Autodesk Fusion 360 part; units mm, degrees
(part 6 of 7)
  spline S1657 degree 3 poles (86.8184, 41.7868) (87.2048, 41.4005) (87.7289, 41.1836) (88.2752, 41.1837) knots 0 0 0 0 1 1 1 1
  spline S1658 degree 3 poles (88.2752, 41.1837) (88.4551, 41.1837) (88.6342, 41.2074) (88.808, 41.254) knots 0 0 0 0 1 1 1 1
  spline S1659 degree 3 poles (88.808, 41.254) (88.982, 41.3005) (89.1491, 41.3696) (89.3051, 41.4596) knots 0 0 0 0 1 1 1 1
  spline S1660 degree 3 poles (89.732, 41.7868) (89.8592, 41.9141) (89.9692, 42.0576) (90.0591, 42.2136) knots 0 0 0 0 1 1 1 1
  spline S1661 degree 3 poles (102.4717, 50.3743) (102.7932, 50.3631) (103.0962, 50.5243) (103.2665, 50.7971) knots 0 0 0 0 1 1 1 1
  line L713 (100.8884, 39.3822) -> (100.8884, 39.3822)
  spline S1662 degree 3 poles (13.6891, 79.1943) (13.7972, 79.0862) (13.8906, 78.9644) (13.9671, 78.832) knots 0 0 0 0 1 1 1 1
  spline S1663 degree 3 poles (100.5907, 54.2211) (100.8269, 53.9847) (101.1474, 53.8518) (101.4816, 53.8516) knots 0 0 0 0 1 1 1 1
  spline S1664 degree 3 poles (102.7415, 55.112) (102.7415, 55.2442) (102.7208, 55.3755) (102.68, 55.5012) knots 0 0 0 0 1 1 1 1
  line L714 (101.4816, 56.3719) -> (101.4816, 56.3719)
  spline S1665 degree 3 poles (99.8394, 34.8063) (99.6692, 34.5338) (99.6572, 34.1914) (99.8078, 33.9076) knots 0 0 0 0 1 1 1 1
  spline S1666 degree 3 poles (103.2981, 51.6962) (103.1471, 51.9801) (102.8562, 52.162) (102.5348, 52.1732) knots 0 0 0 0 1 1 1 1
  spline S1667 degree 3 poles (99.6285, 38.1224) (99.6285, 37.7882) (99.7612, 37.4678) (99.9975, 37.2315) knots 0 0 0 0 1 1 1 1
  spline S1668 degree 3 poles (99.9975, 39.0133) (99.7612, 38.777) (99.6285, 38.4565) (99.6285, 38.1224) knots 0 0 0 0 1 1 1 1
  spline S1669 degree 3 poles (108.2218, 49.423) (108.0708, 49.7069) (107.7799, 49.8887) (107.4585, 49.8999) knots 0 0 0 0 1 1 1 1
  line L715 (102.5348, 52.1732) -> (101.2258, 52.2192)
  spline S1670 degree 3 poles (107.3955, 48.1011) (107.7169, 48.0899) (108.0199, 48.251) (108.1903, 48.5238) knots 0 0 0 0 1 1 1 1
  spline S1671 degree 3 poles (101.6289, 39.1414) (101.5221, 39.2192) (101.4037, 39.2798) (101.278, 39.3208) knots 0 0 0 0 1 1 1 1
  spline S1672 degree 3 poles (100.6321, 35.2295) (100.3113, 35.2399) (100.0092, 35.0786) (99.8394, 34.8063) knots 0 0 0 0 1 1 1 1
  spline S1673 degree 3 poles (102.68, 55.5012) (102.6392, 55.6269) (102.5789, 55.7455) (102.5012, 55.8526) knots 0 0 0 0 1 1 1 1
  spline S1674 degree 3 poles (101.2258, 52.2192) (100.9044, 52.2304) (100.6014, 52.0693) (100.431, 51.7965) knots 0 0 0 0 1 1 1 1
  spline S1675 degree 3 poles (88.808, 45.2336) (88.6342, 45.2802) (88.4551, 45.3038) (88.2752, 45.3038) knots 0 0 0 0 1 1 1 1
  spline S1676 degree 3 poles (102.5012, 55.8526) (102.4234, 55.9595) (102.3292, 56.0535) (102.2222, 56.1311) knots 0 0 0 0 1 1 1 1
  spline S1677 degree 3 poles (88.2752, 45.3038) (87.7288, 45.3038) (87.2048, 45.0867) (86.8184, 44.7003) knots 0 0 0 0 1 1 1 1
  spline S1678 degree 3 poles (100.3995, 50.8968) (100.5506, 50.6131) (100.8415, 50.4315) (101.1628, 50.4203) knots 0 0 0 0 1 1 1 1
  spline S1679 degree 3 poles (102.3725, 54.2211) (102.6088, 54.4574) (102.7415, 54.7779) (102.7415, 55.112) knots 0 0 0 0 1 1 1 1
  line L716 (107.4585, 49.8999) -> (106.149, 49.9459)
  spline S1680 degree 3 poles (108.1903, 48.5238) (108.3606, 48.7964) (108.3726, 49.1391) (108.2218, 49.423) knots 0 0 0 0 1 1 1 1
  spline S1681 degree 3 poles (100.431, 51.7965) (100.2605, 51.5238) (100.2485, 51.1808) (100.3995, 50.8968) knots 0 0 0 0 1 1 1 1
  line L717 (101.1628, 50.4203) -> (102.4717, 50.3743)
  line L718 (101.9416, 35.1835) -> (100.6321, 35.2295)
  spline S1682 degree 3 poles (13.3268, 79.4723) (13.4592, 79.3958) (13.581, 79.3024) (13.6891, 79.1943) knots 0 0 0 0 1 1 1 1
  spline S1683 degree 3 poles (101.7793, 37.2315) (102.0155, 37.4678) (102.1483, 37.7882) (102.1483, 38.1224) knots 0 0 0 0 1 1 1 1
  spline S1684 degree 3 poles (102.6717, 33.8079) (102.8417, 34.0802) (102.8537, 34.4225) (102.7033, 34.706) knots 0 0 0 0 1 1 1 1
  spline S1685 degree 3 poles (101.8713, 56.3104) (101.7454, 56.3512) (101.6139, 56.372) (101.4816, 56.3719) knots 0 0 0 0 1 1 1 1
  line L719 (106.0865, 48.1471) -> (107.3955, 48.1011)
  spline S1686 degree 3 poles (7.9044, 27.4543) (7.5762, 27.1261) (7.3918, 26.6809) (7.3918, 26.2166) knots 0 0 0 0 1 1 1 1
  spline S1687 degree 3 poles (10.3792, 27.4543) (10.2711, 27.5624) (10.1493, 27.6559) (10.017, 27.7323) knots 0 0 0 0 1 1 1 1
  line L720 (89.7935, 43.7174) -> (89.809, 44.6)
  spline S1688 degree 3 poles (4.2705, 32.7832) (4.5987, 32.4552) (5.0437, 32.271) (5.5077, 32.2711) knots 0 0 0 0 1 1 1 1
  spline S1689 degree 3 poles (90.0591, 42.2136) (90.149, 42.3694) (90.2182, 42.5364) (90.2647, 42.7102) knots 0 0 0 0 1 1 1 1
  spline S1690 degree 3 poles (5.5077, 32.2711) (5.9718, 32.2709) (6.417, 32.4551) (6.7453, 32.7832) knots 0 0 0 0 1 1 1 1
  spline S1691 degree 3 poles (4.2705, 35.2585) (3.9423, 34.9302) (3.7579, 34.485) (3.7579, 34.0208) knots 0 0 0 0 1 1 1 1
  spline S1692 degree 3 poles (3.7579, 34.0208) (3.7579, 33.5566) (3.9423, 33.1114) (4.2705, 32.7832) knots 0 0 0 0 1 1 1 1
  spline S1693 degree 3 poles (7.0233, 34.8957) (6.9469, 35.0283) (6.8535, 35.1502) (6.7453, 35.2585) knots 0 0 0 0 1 1 1 1
  line L721 (13.8684, 45.3834) -> (12.5636, 45.2692)
  spline S1694 degree 3 poles (14.0255, 43.5903) (14.3453, 43.6188) (14.6257, 43.8155) (14.7614, 44.1065) knots 0 0 0 0 1 1 1 1
  spline S1695 degree 3 poles (90.2647, 42.7102) (90.3114, 42.8841) (90.335, 43.0634) (90.335, 43.2435) knots 0 0 0 0 1 1 1 1
  spline S1696 degree 3 poles (10.8319, 26.6698) (10.7924, 26.8176) (10.7336, 26.9596) (10.6572, 27.092) knots 0 0 0 0 1 1 1 1
  spline S1697 degree 3 poles (11.9057, 43.8569) (12.0898, 43.5937) (12.4002, 43.4486) (12.7201, 43.4761) knots 0 0 0 0 1 1 1 1
  spline S1698 degree 3 poles (7.258, 34.0208) (7.2578, 34.1737) (7.2377, 34.3259) (7.198, 34.4735) knots 0 0 0 0 1 1 1 1
  line L722 (12.7201, 43.4761) -> (14.0255, 43.5903)
  spline S1699 degree 3 poles (9.1416, 24.4669) (9.6058, 24.4668) (10.051, 24.6512) (10.3792, 24.9795) knots 0 0 0 0 1 1 1 1
  line L723 (26.3307, 38.0412) -> (25.9297, 42.6239)
  spline S1700 degree 3 poles (10.017, 27.7323) (9.8845, 27.8087) (9.7425, 27.8675) (9.5948, 27.907) knots 0 0 0 0 1 1 1 1
  line L724 (25.9297, 42.6239) -> (28.4799, 42.8472)
  spline S1701 degree 3 poles (100.2218, 55.112) (100.2218, 54.7779) (100.3545, 54.4574) (100.5907, 54.2211) knots 0 0 0 0 1 1 1 1
  line L725 (28.438, 43.3252) -> (28.9109, 43.8884)
  spline S1702 degree 3 poles (44.1058, 40.5264) (43.9601, 40.2401) (43.978, 39.8978) (44.1528, 39.6282) knots 0 0 0 0 1 1 1 1
  spline S1703 degree 3 poles (44.1528, 39.6282) (44.3277, 39.359) (44.6327, 39.2032) (44.9533, 39.2195) knots 0 0 0 0 1 1 1 1
  spline S1704 degree 3 poles (9.5948, 27.907) (9.447, 27.9467) (9.2946, 27.9668) (9.1416, 27.9669) knots 0 0 0 0 1 1 1 1
  line L726 (90.2735, 43.7091) -> (89.7935, 43.7174)
  spline S1705 degree 3 poles (6.7453, 35.2585) (6.6371, 35.3666) (6.5151, 35.4601) (6.3826, 35.5365) knots 0 0 0 0 1 1 1 1
  spline S1706 degree 3 poles (7.198, 34.4735) (7.1585, 34.6213) (7.0998, 34.7632) (7.0233, 34.8957) knots 0 0 0 0 1 1 1 1
  spline S1707 degree 3 poles (12.5636, 45.2692) (12.2434, 45.2408) (11.9628, 45.0438) (11.8272, 44.7525) knots 0 0 0 0 1 1 1 1
  spline S1708 degree 3 poles (100.5907, 56.0029) (100.3545, 55.7666) (100.2218, 55.4462) (100.2218, 55.112) knots 0 0 0 0 1 1 1 1
  spline S1709 degree 3 poles (32.9866, 37.386) (32.6898, 37.5925) (32.3263, 37.6801) (31.9681, 37.6315) knots 0 0 0 0 1 1 1 1
  spline S1710 degree 3 poles (89.3051, 41.4596) (89.4611, 41.5496) (89.6046, 41.6595) (89.732, 41.7868) knots 0 0 0 0 1 1 1 1
  line L727 (44.9533, 39.2195) -> (46.2612, 39.2877)
  line L728 (28.9109, 43.8884) -> (33.892, 44.3246)
  line L729 (30.3738, 37.4919) -> (29.3491, 38.3053)
  line L730 (46.1672, 41.0855) -> (44.8593, 41.0168)
  line L731 (31.9681, 37.6315) -> (30.3738, 37.4919)
  spline S1711 degree 3 poles (7.3918, 26.2166) (7.3919, 25.7526) (7.5763, 25.3076) (7.9044, 24.9795) knots 0 0 0 0 1 1 1 1
  spline S1712 degree 3 poles (46.2612, 39.2877) (46.582, 39.3051) (46.8691, 39.4922) (47.0147, 39.7786) knots 0 0 0 0 1 1 1 1
  spline S1713 degree 3 poles (7.9044, 24.9795) (8.2325, 24.6514) (8.6775, 24.467) (9.1416, 24.4669) knots 0 0 0 0 1 1 1 1
  spline S1714 degree 3 poles (46.9677, 40.6762) (46.793, 40.9457) (46.4879, 41.1017) (46.1672, 41.0855) knots 0 0 0 0 1 1 1 1
  spline S1715 degree 3 poles (9.1416, 27.9669) (8.6775, 27.9668) (8.2325, 27.7824) (7.9044, 27.4543) knots 0 0 0 0 1 1 1 1
  spline S1716 degree 3 poles (33.5711, 36.5168) (33.4919, 36.8695) (33.2834, 37.1796) (32.9866, 37.386) knots 0 0 0 0 1 1 1 1
  spline S1717 degree 3 poles (6.7453, 32.7832) (7.0736, 33.1114) (7.258, 33.5566) (7.258, 34.0208) knots 0 0 0 0 1 1 1 1
  spline S1718 degree 3 poles (90.335, 43.2435) (90.3323, 43.4005) (90.3117, 43.5568) (90.2735, 43.7091) knots 0 0 0 0 1 1 1 1
  line L732 (46.1672, 41.0855) -> (46.1672, 41.0855)
  line L733 (28.4799, 42.8472) -> (28.438, 43.3252)
  spline S1719 degree 3 poles (10.3792, 24.9795) (10.7073, 25.3076) (10.8917, 25.7526) (10.8918, 26.2166) knots 0 0 0 0 1 1 1 1
  spline S1720 degree 3 poles (5.5077, 35.7706) (5.0437, 35.7706) (4.5987, 35.5864) (4.2705, 35.2585) knots 0 0 0 0 1 1 1 1
  spline S1721 degree 3 poles (10.6572, 27.092) (10.5808, 27.2244) (10.4873, 27.3462) (10.3792, 27.4543) knots 0 0 0 0 1 1 1 1
  spline S1722 degree 3 poles (6.3826, 35.5365) (6.2502, 35.6129) (6.1085, 35.6716) (5.9609, 35.7112) knots 0 0 0 0 1 1 1 1
  spline S1723 degree 3 poles (11.8272, 44.7525) (11.6917, 44.4613) (11.7217, 44.12) (11.9057, 43.8569) knots 0 0 0 0 1 1 1 1
  spline S1724 degree 3 poles (10.8918, 26.2166) (10.8918, 26.3697) (10.8716, 26.5221) (10.8319, 26.6698) knots 0 0 0 0 1 1 1 1
  line L734 (29.3491, 38.3053) -> (26.3307, 38.0412)
  line L735 (9.1416, 27.9669) -> (9.1416, 27.9669)
  spline S1725 degree 3 poles (5.9609, 35.7112) (5.8131, 35.7507) (5.6607, 35.7707) (5.5077, 35.7706) knots 0 0 0 0 1 1 1 1
  spline S1726 degree 3 poles (44.8593, 41.0168) (44.5386, 40.9994) (44.2515, 40.8125) (44.1058, 40.5264) knots 0 0 0 0 1 1 1 1
  line L736 (8.7044, 47.0397) -> (7.3995, 46.9255)
  line L737 (5.5077, 35.7706) -> (5.5077, 35.7706)
  spline S1727 degree 3 poles (9.5973, 45.7627) (9.733, 46.054) (9.7031, 46.3956) (9.5188, 46.6588) knots 0 0 0 0 1 1 1 1
  line L738 (7.5561, 45.1323) -> (8.8615, 45.2465)
  spline S1728 degree 3 poles (46.2457, 41.086) (46.5388, 41.0752) (46.8081, 40.9223) (46.9677, 40.6762) knots 0 0 0 0 1 1 1 1
  spline S1729 degree 3 poles (9.5188, 46.6588) (9.3347, 46.922) (9.0244, 47.0671) (8.7044, 47.0397) knots 0 0 0 0 1 1 1 1
  spline S1730 degree 3 poles (47.0147, 39.7786) (47.1602, 40.0648) (47.1423, 40.4068) (46.9677, 40.6762) knots 0 0 0 0 1 1 1 1
  spline S1731 degree 3 poles (6.6626, 46.4087) (6.527, 46.1174) (6.5569, 45.7759) (6.7412, 45.5126) knots 0 0 0 0 1 1 1 1
  spline S1732 degree 3 poles (7.3995, 46.9255) (7.0792, 46.8972) (6.7983, 46.7002) (6.6626, 46.4087) knots 0 0 0 0 1 1 1 1
  spline S1733 degree 3 poles (6.7412, 45.5126) (6.9255, 45.2495) (7.2361, 45.1045) (7.5561, 45.1323) knots 0 0 0 0 1 1 1 1
  spline S1734 degree 3 poles (8.8615, 45.2465) (9.1813, 45.275) (9.4617, 45.4717) (9.5973, 45.7627) knots 0 0 0 0 1 1 1 1
  spline S1735 degree 3 poles (44.9533, 39.2195) (44.6327, 39.2032) (44.3277, 39.359) (44.1528, 39.6282) knots 0 0 0 0 1 1 1 1
  line L739 (8.7044, 47.0397) -> (8.7044, 47.0397)
  spline S1736 degree 3 poles (44.1058, 40.5264) (44.2515, 40.8125) (44.5386, 40.9994) (44.8593, 41.0168) knots 0 0 0 0 1 1 1 1
  spline S1737 degree 3 poles (44.1528, 39.6282) (43.978, 39.8978) (43.9601, 40.2401) (44.1058, 40.5264) knots 0 0 0 0 1 1 1 1
  spline S1738 degree 3 poles (13.9469, 45.3865) (14.2401, 45.386) (14.5147, 45.2428) (14.6828, 45.0026) knots 0 0 0 0 1 1 1 1
  line L740 (46.2457, 41.086) -> (46.2457, 41.086)
  spline S1739 degree 3 poles (14.6828, 45.0026) (14.8671, 44.7393) (14.897, 44.3978) (14.7614, 44.1065) knots 0 0 0 0 1 1 1 1
  spline S1740 degree 3 poles (46.1672, 41.0855) (46.1934, 41.0868) (46.2196, 41.087) (46.2457, 41.086) knots 0 0 0 0 1 1 1 1
  spline S1741 degree 3 poles (12.7201, 43.4761) (12.4002, 43.4486) (12.0898, 43.5937) (11.9057, 43.8569) knots 0 0 0 0 1 1 1 1
  line L741 (44.8593, 41.0168) -> (46.1672, 41.0855)
  spline S1742 degree 3 poles (14.7614, 44.1065) (14.6257, 43.8155) (14.3453, 43.6188) (14.0255, 43.5903) knots 0 0 0 0 1 1 1 1
  line L742 (14.0255, 43.5903) -> (12.7201, 43.4761)
  spline S1743 degree 3 poles (46.9677, 40.6762) (47.1423, 40.4068) (47.1602, 40.0648) (47.0147, 39.7786) knots 0 0 0 0 1 1 1 1
  spline S1744 degree 3 poles (47.0147, 39.7786) (46.8691, 39.4922) (46.582, 39.3051) (46.2612, 39.2877) knots 0 0 0 0 1 1 1 1
  line L743 (46.2612, 39.2877) -> (44.9533, 39.2195)
  line L744 (70.0851, 82.9434) -> (68.4852, 82.9434)
  spline S1745 degree 3 poles (59.9705, 77.2166) (59.5755, 77.2167) (59.1875, 77.3208) (58.8455, 77.5184) knots 0 0 0 0 1 1 1 1
  spline S1746 degree 3 poles (71.5853, 81.6933) (71.5371, 82.0518) (71.3562, 82.3791) (71.0783, 82.6106) knots 0 0 0 0 1 1 1 1
  spline S1747 degree 3 poles (68.6185, 78.7871) (68.2321, 79.1734) (68.015, 79.6974) (68.0149, 80.2438) knots 0 0 0 0 1 1 1 1
  spline S1748 degree 3 poles (68.6185, 81.7001) (69.0048, 82.0865) (69.5289, 82.3036) (70.0753, 82.3036) knots 0 0 0 0 1 1 1 1
  spline S1749 degree 3 poles (70.3523, 89.4438) (70.5558, 89.5244) (70.7726, 89.5661) (70.9915, 89.5668) knots 0 0 0 0 1 1 1 1
  spline S1750 degree 3 poles (61.9187, 78.3416) (61.7213, 77.9997) (61.4373, 77.7158) (61.0955, 77.5184) knots 0 0 0 0 1 1 1 1
  spline S1751 degree 3 poles (58.8455, 77.5184) (58.5034, 77.7158) (58.2193, 77.9997) (58.0218, 78.3416) knots 0 0 0 0 1 1 1 1
  spline S1752 degree 3 poles (70.0753, 82.3036) (70.2552, 82.3036) (70.4343, 82.28) (70.6081, 82.2334) knots 0 0 0 0 1 1 1 1
  line L745 (56.4983, 80.0294) -> (56.548, 79.0806)
  line L746 (58.8289, 84.7578) -> (59.0021, 81.4572)
  spline S1753 degree 3 poles (59.0021, 81.4572) (59.3013, 81.6154) (59.6323, 81.7041) (59.9705, 81.7166) knots 0 0 0 0 1 1 1 1
  spline S1754 degree 3 poles (60.4707, 81.6603) (60.6351, 81.6228) (60.7947, 81.567) (60.9466, 81.4939) knots 0 0 0 0 1 1 1 1
  spline S1755 degree 3 poles (55.1796, 79.0088) (55.2126, 78.9545) (55.2414, 78.8979) (55.2659, 78.8393) knots 0 0 0 0 1 1 1 1
  spline S1756 degree 3 poles (55.2659, 78.8393) (55.3066, 78.7136) (55.3274, 78.5823) (55.3274, 78.4501) knots 0 0 0 0 1 1 1 1
  spline S1757 degree 3 poles (54.9584, 77.5592) (54.7222, 77.3228) (54.4017, 77.1899) (54.0675, 77.1897) knots 0 0 0 0 1 1 1 1
  spline S1758 degree 3 poles (55.3274, 78.4501) (55.3274, 78.116) (55.1946, 77.7955) (54.9584, 77.5592) knots 0 0 0 0 1 1 1 1
  spline S1759 degree 3 poles (70.0753, 78.1835) (69.5289, 78.1835) (69.0048, 78.4006) (68.6185, 78.7871) knots 0 0 0 0 1 1 1 1
  spline S1760 degree 3 poles (54.0675, 77.1897) (53.7333, 77.1899) (53.4128, 77.3228) (53.1766, 77.5592) knots 0 0 0 0 1 1 1 1
  spline S1761 degree 3 poles (50.5359, 78.7654) (50.546, 78.7421) (50.5556, 78.7187) (50.5649, 78.6951) knots 0 0 0 0 1 1 1 1
  spline S1762 degree 3 poles (52.8076, 78.4501) (52.8399, 78.6085) (52.9023, 78.7592) (52.9916, 78.894) knots 0 0 0 0 1 1 1 1
  spline S1763 degree 3 poles (50.5649, 78.6951) (50.6114, 78.5213) (50.6351, 78.3422) (50.6351, 78.1623) knots 0 0 0 0 1 1 1 1
  line L747 (52.9916, 78.894) -> (50.5359, 78.7654)
  spline S1764 degree 3 poles (50.6351, 78.1623) (50.6351, 77.9822) (50.6115, 77.8029) (50.5649, 77.629) knots 0 0 0 0 1 1 1 1
  line L748 (67.0651, 88.9234) -> (67.585, 89.4438)
  spline S1765 degree 3 poles (51.3416, 85.6621) (51.4403, 85.5732) (51.5707, 85.5278) (51.7033, 85.536) knots 0 0 0 0 1 1 1 1
  spline S1766 degree 3 poles (50.5649, 77.629) (50.5183, 77.455) (50.4492, 77.2879) (50.3592, 77.1319) knots 0 0 0 0 1 1 1 1
  spline S1767 degree 3 poles (50.0316, 76.7055) (49.9044, 76.5782) (49.761, 76.468) (49.6052, 76.3779) knots 0 0 0 0 1 1 1 1
  line L749 (67.585, 89.4438) -> (70.3523, 89.4438)
  line L750 (51.1255, 87.0077) -> (51.1783, 86.0088)
  spline S1768 degree 3 poles (61.7295, 80.8696) (61.8345, 80.7378) (61.9243, 80.5946) (61.9972, 80.4428) knots 0 0 0 0 1 1 1 1
  line L751 (56.1976, 85.7716) -> (56.2575, 84.6229)
  spline S1769 degree 3 poles (53.1766, 77.5592) (52.9403, 77.7955) (52.8076, 78.116) (52.8076, 78.4501) knots 0 0 0 0 1 1 1 1
  line L752 (56.548, 79.0806) -> (55.1796, 79.0088)
  line L753 (71.5853, 81.6303) -> (71.5853, 81.6933)
  line L754 (70.9915, 89.5668) -> (70.9915, 89.5668)
  line L755 (51.7033, 85.536) -> (56.1976, 85.7716)
  spline S1770 degree 3 poles (61.373, 81.2257) (61.5048, 81.1207) (61.6244, 81.0013) (61.7295, 80.8696) knots 0 0 0 0 1 1 1 1
  line L756 (57.8905, 80.1022) -> (56.4983, 80.0294)
  spline S1771 degree 3 poles (59.9705, 81.7166) (60.1388, 81.7166) (60.3066, 81.6977) (60.4707, 81.6603) knots 0 0 0 0 1 1 1 1
  spline S1772 degree 3 poles (71.1052, 82.0277) (71.261, 81.9376) (71.4043, 81.8274) (71.5315, 81.7001) knots 0 0 0 0 1 1 1 1
  spline S1773 degree 3 poles (57.7205, 79.4666) (57.7457, 79.6857) (57.803, 79.8998) (57.8905, 80.1022) knots 0 0 0 0 1 1 1 1
  spline S1774 degree 3 poles (68.0149, 80.2438) (68.0151, 80.7901) (68.2322, 81.3139) (68.6185, 81.7001) knots 0 0 0 0 1 1 1 1
  spline S1775 degree 3 poles (71.0783, 82.6106) (70.8006, 82.842) (70.4462, 82.9607) (70.0851, 82.9434) knots 0 0 0 0 1 1 1 1
  line L757 (64.5051, 88.4438) -> (67.0651, 88.4438)
  spline S1776 degree 3 poles (70.6081, 78.2538) (70.4343, 78.2072) (70.2552, 78.1835) (70.0753, 78.1835) knots 0 0 0 0 1 1 1 1
  spline S1777 degree 3 poles (71.5315, 81.7001) (71.5499, 81.6772) (71.5679, 81.6539) (71.5853, 81.6303) knots 0 0 0 0 1 1 1 1
  line L758 (68.4852, 82.9434) -> (67.5349, 83.8436)
  spline S1778 degree 3 poles (61.9972, 80.4428) (62.0703, 80.291) (62.1261, 80.1316) (62.1636, 79.9674) knots 0 0 0 0 1 1 1 1
  spline S1779 degree 3 poles (62.2205, 79.4666) (62.2204, 79.0716) (62.1163, 78.6836) (61.9187, 78.3416) knots 0 0 0 0 1 1 1 1
  line L759 (64.5051, 83.8436) -> (64.5051, 88.4438)
  spline S1780 degree 3 poles (51.1783, 86.0088) (51.1839, 85.876) (51.2428, 85.7511) (51.3416, 85.6621) knots 0 0 0 0 1 1 1 1
  line L760 (56.2575, 84.6229) -> (58.8289, 84.7578)
  spline S1781 degree 3 poles (60.9466, 81.4939) (61.0983, 81.4207) (61.2414, 81.3307) (61.373, 81.2257) knots 0 0 0 0 1 1 1 1
  spline S1782 degree 3 poles (70.6081, 82.2334) (70.7821, 82.1868) (70.9492, 82.1177) (71.1052, 82.0277) knots 0 0 0 0 1 1 1 1
  spline S1783 degree 3 poles (62.1636, 79.9674) (62.2013, 79.8031) (62.2203, 79.6351) (62.2205, 79.4666) knots 0 0 0 0 1 1 1 1
  line L761 (50.6, 87.4811) -> (51.1255, 87.0077)
  spline S1784 degree 3 poles (61.0955, 77.5184) (60.7535, 77.3208) (60.3655, 77.2167) (59.9705, 77.2166) knots 0 0 0 0 1 1 1 1
  line L762 (67.0651, 88.4438) -> (67.0651, 88.9234)
  spline S1785 degree 3 poles (58.0218, 78.3416) (57.8243, 78.6837) (57.7204, 79.0717) (57.7205, 79.4666) knots 0 0 0 0 1 1 1 1
  line L763 (67.5349, 83.8436) -> (64.5051, 83.8436)
  line L764 (91.5386, 86.3933) -> (92.03, 85.8843)
  spline S1786 degree 3 poles (46.515, 78.1623) (46.5151, 78.7085) (46.7322, 79.2323) (47.1186, 79.6185) knots 0 0 0 0 1 1 1 1
  line L765 (46.8462, 80.7751) -> (45.8504, 81.6241)
  line L766 (45.8504, 81.6241) -> (42.8242, 81.4655)
  line L767 (48.4441, 80.8588) -> (46.8462, 80.7751)
  spline S1787 degree 3 poles (92.0124, 84.8849) (92.0087, 84.7519) (92.0586, 84.623) (92.1509, 84.5273) knots 0 0 0 0 1 1 1 1
  line L768 (96.9026, 78.5483) -> (96.886, 77.5985)
  spline S1788 degree 3 poles (49.6052, 76.3779) (49.4492, 76.2879) (49.2821, 76.2188) (49.1081, 76.1722) knots 0 0 0 0 1 1 1 1
  spline S1789 degree 3 poles (49.6052, 79.9462) (49.7525, 79.8596) (49.8884, 79.7551) (50.0099, 79.6351) knots 0 0 0 0 1 1 1 1
  line L769 (99.4771, 78.5034) -> (96.9026, 78.5483)
  line L770 (99.5572, 83.1026) -> (99.4771, 78.5034)
  spline S1790 degree 3 poles (95.6277, 77.1422) (95.6277, 76.8081) (95.495, 76.4876) (95.2588, 76.2513) knots 0 0 0 0 1 1 1 1
  line L771 (93.3219, 77.661) -> (90.8673, 77.7039)
  line L772 (72.5852, 89.4438) -> (73.0849, 88.9435)
  spline S1791 degree 3 poles (50.0073, 79.6893) (49.9404, 80.0445) (49.7427, 80.3617) (49.4533, 80.5782) knots 0 0 0 0 1 1 1 1
  spline S1792 degree 3 poles (70.9915, 89.5668) (71.1445, 89.5669) (71.2969, 89.5469) (71.4447, 89.5073) knots 0 0 0 0 1 1 1 1
  line L773 (42.8242, 81.4655) -> (42.5834, 86.0595)
  spline S1793 degree 3 poles (48.5753, 80.2221) (48.7552, 80.2221) (48.9343, 80.1984) (49.1081, 80.1518) knots 0 0 0 0 1 1 1 1
  line L774 (45.607, 87.2191) -> (50.6, 87.4811)
  line L775 (50.0099, 79.6351) -> (50.0073, 79.6893)
  line L776 (73.0849, 88.9435) -> (73.0849, 87.9436)
  line L777 (69.4722, 91.2426) -> (69.4722, 91.2426)
  spline S1794 degree 3 poles (71.4447, 89.5073) (71.508, 89.4897) (71.5703, 89.4685) (71.6313, 89.4438) knots 0 0 0 0 1 1 1 1
  line L778 (78.0851, 87.4434) -> (78.0851, 86.2936)
  line L779 (80.6602, 86.2936) -> (80.6602, 81.6933)
  spline S1795 degree 3 poles (94.3679, 75.8823) (94.0335, 75.8822) (93.7129, 76.0149) (93.4764, 76.2513) knots 0 0 0 0 1 1 1 1
  spline S1796 degree 3 poles (48.5753, 76.102) (48.0289, 76.102) (47.5049, 76.3191) (47.1186, 76.7055) knots 0 0 0 0 1 1 1 1
  spline S1797 degree 3 poles (49.4533, 80.5782) (49.1639, 80.7948) (48.8037, 80.8949) (48.4441, 80.8588) knots 0 0 0 0 1 1 1 1
  spline S1798 degree 3 poles (92.1509, 84.5273) (92.2433, 84.4315) (92.3703, 84.3769) (92.5034, 84.3759) knots 0 0 0 0 1 1 1 1
  spline S1799 degree 3 poles (50.3592, 77.1319) (50.2691, 76.9761) (50.1589, 76.8327) (50.0316, 76.7055) knots 0 0 0 0 1 1 1 1
  spline S1800 degree 3 poles (47.1186, 76.7055) (46.7321, 77.0919) (46.515, 77.6159) (46.515, 78.1623) knots 0 0 0 0 1 1 1 1
  line L780 (45.1399, 86.1933) -> (45.1151, 86.6729)
  line L781 (92.5034, 84.3759) -> (97.0028, 84.2973)
  spline S1801 degree 3 poles (47.1186, 79.6185) (47.5049, 80.005) (48.0289, 80.2221) (48.5753, 80.2221) knots 0 0 0 0 1 1 1 1
  line L782 (86.5394, 86.4807) -> (91.5386, 86.3933)
  spline S1802 degree 3 poles (95.5197, 77.6223) (95.5363, 77.5928) (95.5516, 77.5626) (95.5657, 77.5318) knots 0 0 0 0 1 1 1 1
  line L783 (92.03, 85.8843) -> (92.0124, 84.8849)
  line L784 (96.886, 77.5985) -> (95.5197, 77.6223)
  spline S1803 degree 3 poles (93.1075, 77.1422) (93.139, 77.3291) (93.2123, 77.5064) (93.3219, 77.661) knots 0 0 0 0 1 1 1 1
  spline S1804 degree 3 poles (90.9283, 77.2383) (90.9284, 77.0583) (90.905, 76.879) (90.8585, 76.705) knots 0 0 0 0 1 1 1 1
  line L785 (42.5834, 86.0595) -> (45.1399, 86.1933)
  spline S1805 degree 3 poles (95.5657, 77.5318) (95.6067, 77.406) (95.6276, 77.2745) (95.6277, 77.1422) knots 0 0 0 0 1 1 1 1
  spline S1806 degree 3 poles (49.1081, 76.1722) (48.9343, 76.1256) (48.7552, 76.102) (48.5753, 76.102) knots 0 0 0 0 1 1 1 1
  line L786 (96.9827, 83.1475) -> (99.5572, 83.1026)
  spline S1807 degree 3 poles (95.2588, 76.2513) (95.0225, 76.015) (94.702, 75.8823) (94.3679, 75.8823) knots 0 0 0 0 1 1 1 1
  spline S1808 degree 3 poles (93.4764, 76.2513) (93.2402, 76.4876) (93.1075, 76.8081) (93.1075, 77.1422) knots 0 0 0 0 1 1 1 1
  spline S1809 degree 3 poles (49.1081, 80.1518) (49.2821, 80.1053) (49.4492, 80.0362) (49.6052, 79.9462) knots 0 0 0 0 1 1 1 1
  spline S1810 degree 3 poles (90.8673, 77.7039) (90.9053, 77.5516) (90.9258, 77.3953) (90.9283, 77.2383) knots 0 0 0 0 1 1 1 1
  line L787 (71.6313, 89.4438) -> (72.5852, 89.4438)
  spline S1811 degree 3 poles (77.7751, 91.0954) (75.0088, 91.2019) (72.2406, 91.251) (69.4722, 91.2426) knots 0 0 0 0 1 1 1 1
  line L788 (78.0851, 86.2936) -> (80.6602, 86.2936)
  line L789 (45.1151, 86.6729) -> (45.607, 87.2191)
  line L790 (97.0028, 84.2973) -> (96.9827, 83.1475)
  line L791 (73.5851, 87.4434) -> (78.0851, 87.4434)
  spline S1812 degree 3 poles (91.1743, 16.8741) (90.9637, 16.6315) (90.8983, 16.2952) (91.0027, 15.9914) knots 0 0 0 0 1 1 1 1
  line L792 (78.0851, 81.6933) -> (78.0851, 80.7435)
  spline S1813 degree 3 poles (76.7736, 80.6329) (76.8144, 80.5073) (76.8351, 80.376) (76.8351, 80.2438) knots 0 0 0 0 1 1 1 1
  spline S1814 degree 3 poles (76.8351, 80.2438) (76.8352, 79.9095) (76.7025, 79.5888) (76.4661, 79.3524) knots 0 0 0 0 1 1 1 1
  line L793 (74.522, 80.7435) -> (72.069, 80.7435)
  spline S1815 degree 3 poles (102.6366, 16.995) (102.4002, 17.2312) (102.2672, 17.5517) (102.2671, 17.8859) knots 0 0 0 0 1 1 1 1
  spline S1816 degree 3 poles (95.6815, 13.8587) (95.4709, 13.6162) (95.4055, 13.2799) (95.5099, 12.9761) knots 0 0 0 0 1 1 1 1
  spline S1817 degree 3 poles (72.0648, 79.7105) (72.0183, 79.5365) (71.9492, 79.3694) (71.8592, 79.2134) knots 0 0 0 0 1 1 1 1
  spline S1818 degree 3 poles (104.7874, 17.8859) (104.7874, 17.5517) (104.6547, 17.2313) (104.4184, 16.995) knots 0 0 0 0 1 1 1 1
  line L794 (78.0851, 80.7435) -> (76.7173, 80.7435)
  spline S1819 degree 3 poles (99.9122, 19.9654) (99.8223, 20.1213) (99.7123, 20.2648) (99.5851, 20.3922) knots 0 0 0 0 1 1 1 1
  line L795 (96.1879, 12.3855) -> (97.4736, 12.1353)
  spline S1820 degree 3 poles (73.2301, 87.5886) (73.3241, 87.4944) (73.4521, 87.4421) (73.5851, 87.4434) knots 0 0 0 0 1 1 1 1
  spline S1821 degree 3 poles (71.8592, 79.2134) (71.769, 79.0576) (71.6589, 78.9143) (71.5315, 78.7871) knots 0 0 0 0 1 1 1 1
  spline S1822 degree 3 poles (74.3148, 80.2438) (74.3469, 80.4234) (74.4176, 80.5939) (74.522, 80.7435) knots 0 0 0 0 1 1 1 1
  spline S1823 degree 3 poles (72.1351, 80.2438) (72.1351, 80.0637) (72.1115, 79.8845) (72.0648, 79.7105) knots 0 0 0 0 1 1 1 1
  spline S1824 degree 3 poles (104.5466, 18.6264) (104.6244, 18.5194) (104.6849, 18.4008) (104.7259, 18.275) knots 0 0 0 0 1 1 1 1
  spline S1825 degree 3 poles (103.5275, 16.626) (103.1934, 16.626) (102.8729, 16.7587) (102.6366, 16.995) knots 0 0 0 0 1 1 1 1
  spline S1826 degree 3 poles (72.069, 80.7435) (72.1114, 80.5803) (72.1336, 80.4125) (72.1351, 80.2438) knots 0 0 0 0 1 1 1 1
  spline S1827 degree 3 poles (96.5315, 14.1523) (96.2161, 14.2132) (95.8921, 14.1013) (95.6815, 13.8587) knots 0 0 0 0 1 1 1 1
  spline S1828 degree 3 poles (97.4736, 12.1353) (97.7888, 12.075) (98.1123, 12.187) (98.3226, 12.4294) knots 0 0 0 0 1 1 1 1
  spline S1829 degree 3 poles (99.5851, 20.3922) (99.4577, 20.5194) (99.3142, 20.6294) (99.1583, 20.7193) knots 0 0 0 0 1 1 1 1
  spline S1830 degree 3 poles (98.4937, 13.3115) (98.3896, 13.6148) (98.1319, 13.8399) (97.8173, 13.9022) knots 0 0 0 0 1 1 1 1
  spline S1831 degree 3 poles (91.0027, 15.9914) (91.1071, 15.6877) (91.3655, 15.4626) (91.6807, 15.4008) knots 0 0 0 0 1 1 1 1
  line L796 (98.1283, 20.9953) -> (98.1283, 20.9953)
  line L797 (91.6807, 15.4008) -> (92.9664, 15.1507)
  spline S1832 degree 3 poles (99.1583, 20.7193) (99.0024, 20.8093) (98.8355, 20.8784) (98.6616, 20.925) knots 0 0 0 0 1 1 1 1
  spline S1833 degree 3 poles (93.9891, 16.3273) (93.8843, 16.6312) (93.6255, 16.8561) (93.31, 16.9175) knots 0 0 0 0 1 1 1 1
  spline S1834 degree 3 poles (104.268, 18.9055) (104.3749, 18.8276) (104.4689, 18.7335) (104.5466, 18.6264) knots 0 0 0 0 1 1 1 1
  spline S1835 degree 3 poles (76.7173, 80.7435) (76.7378, 80.7076) (76.7566, 80.6707) (76.7736, 80.6329) knots 0 0 0 0 1 1 1 1
  spline S1836 degree 3 poles (104.4184, 16.995) (104.1821, 16.7587) (103.8616, 16.626) (103.5275, 16.626) knots 0 0 0 0 1 1 1 1
  spline S1837 degree 3 poles (98.3226, 12.4294) (98.5329, 12.6719) (98.598, 13.008) (98.4937, 13.3115) knots 0 0 0 0 1 1 1 1
  spline S1838 degree 3 poles (76.4661, 79.3524) (76.2298, 79.1162) (75.9094, 78.9834) (75.5752, 78.9834) knots 0 0 0 0 1 1 1 1
  spline S1839 degree 3 poles (92.0238, 17.1676) (91.7085, 17.2283) (91.3848, 17.1164) (91.1743, 16.8741) knots 0 0 0 0 1 1 1 1
  spline S1840 degree 3 poles (73.0849, 87.9436) (73.0836, 87.8106) (73.136, 87.6826) (73.2301, 87.5886) knots 0 0 0 0 1 1 1 1
  spline S1841 degree 3 poles (74.6843, 79.3524) (74.4477, 79.5887) (74.3148, 79.9094) (74.3148, 80.2438) knots 0 0 0 0 1 1 1 1
  spline S1842 degree 3 poles (98.6616, 20.925) (98.4877, 20.9716) (98.3084, 20.9952) (98.1283, 20.9953) knots 0 0 0 0 1 1 1 1
  spline S1843 degree 3 poles (104.7259, 18.275) (104.7666, 18.1493) (104.7874, 18.018) (104.7874, 17.8859) knots 0 0 0 0 1 1 1 1
  spline S1844 degree 3 poles (75.5752, 78.9834) (75.2411, 78.9834) (74.9206, 79.1162) (74.6843, 79.3524) knots 0 0 0 0 1 1 1 1
  spline S1845 degree 3 poles (71.1052, 78.4594) (70.9492, 78.3694) (70.7821, 78.3003) (70.6081, 78.2538) knots 0 0 0 0 1 1 1 1
  spline S1846 degree 3 poles (95.5099, 12.9761) (95.6143, 12.6723) (95.8727, 12.4472) (96.1879, 12.3855) knots 0 0 0 0 1 1 1 1
  line L798 (97.8173, 13.9022) -> (96.5315, 14.1523)
  line L799 (80.6602, 81.6933) -> (78.0851, 81.6933)
  spline S1847 degree 3 poles (71.5315, 78.7871) (71.4043, 78.6597) (71.261, 78.5496) (71.1052, 78.4594) knots 0 0 0 0 1 1 1 1
  spline S1848 degree 3 poles (91.4693, 19.985) (91.4692, 19.6507) (91.6019, 19.33) (91.8383, 19.0936) knots 0 0 0 0 1 1 1 1
  spline S1849 degree 3 poles (92.9664, 15.1507) (93.2821, 15.0892) (93.6065, 15.2009) (93.8175, 15.4437) knots 0 0 0 0 1 1 1 1
  spline S1850 degree 3 poles (92.7292, 18.7246) (92.8615, 18.7247) (92.993, 18.7456) (93.1188, 18.7866) knots 0 0 0 0 1 1 1 1
  line L800 (39.3118, 20.7818) -> (86.2118, 20.7818)
  spline S1851 degree 3 poles (91.8383, 19.0936) (92.0746, 18.8573) (92.3951, 18.7246) (92.7292, 18.7246) knots 0 0 0 0 1 1 1 1
  line L801 (86.2118, 38.372) -> (42.5183, 38.372)
  spline S1852 degree 3 poles (93.1188, 18.7866) (93.2446, 18.8274) (93.3632, 18.8877) (93.4702, 18.9654) knots 0 0 0 0 1 1 1 1
  spline S1853 degree 3 poles (92.7292, 21.2449) (92.3951, 21.2449) (92.0746, 21.1121) (91.8383, 20.8759) knots 0 0 0 0 1 1 1 1
  line L802 (42.5183, 38.372) -> (42.6113, 37.3074)
  spline S1854 degree 3 poles (93.4702, 18.9654) (93.5771, 19.0431) (93.6711, 19.1371) (93.7488, 19.2439) knots 0 0 0 0 1 1 1 1
  line L803 (92.7292, 21.2449) -> (92.7292, 21.2449)
  spline S1855 degree 3 poles (93.9276, 19.5953) (93.9686, 19.7212) (93.9895, 19.8527) (93.9896, 19.985) knots 0 0 0 0 1 1 1 1
  line L804 (42.6113, 37.3074) -> (40.0461, 37.0832)
  line L805 (40.0461, 37.0832) -> (40.1293, 36.137)
  line L806 (96.5315, 14.1523) -> (97.8173, 13.9022)
  spline S1856 degree 3 poles (98.3226, 12.4294) (98.1123, 12.187) (97.7888, 12.075) (97.4736, 12.1353) knots 0 0 0 0 1 1 1 1
  line L807 (86.2118, 20.7818) -> (86.2118, 38.372)
  line L808 (39.3118, 36.0657) -> (39.3118, 20.7818)
  spline S1857 degree 3 poles (93.9896, 19.985) (93.9894, 20.1171) (93.9685, 20.2485) (93.9276, 20.3741) knots 0 0 0 0 1 1 1 1
  line L809 (40.1293, 36.137) -> (39.3118, 36.0657)
  spline S1858 degree 3 poles (93.9276, 20.3741) (93.8868, 20.4999) (93.8264, 20.6185) (93.7488, 20.7255) knots 0 0 0 0 1 1 1 1
  spline S1859 degree 3 poles (93.7488, 19.2439) (93.8264, 19.351) (93.8868, 19.4696) (93.9276, 19.5953) knots 0 0 0 0 1 1 1 1
  spline S1860 degree 3 poles (91.8383, 20.8759) (91.602, 20.6396) (91.4693, 20.3191) (91.4693, 19.985) knots 0 0 0 0 1 1 1 1
  line L810 (93.31, 16.9175) -> (92.0238, 17.1676)
  spline S1861 degree 3 poles (97.8173, 13.9022) (98.1319, 13.8399) (98.3896, 13.6148) (98.4937, 13.3115) knots 0 0 0 0 1 1 1 1
  spline S1862 degree 3 poles (96.3755, 14.1683) (96.4279, 14.1675) (96.4801, 14.1621) (96.5315, 14.1523) knots 0 0 0 0 1 1 1 1
  spline S1863 degree 3 poles (98.4937, 13.3115) (98.598, 13.008) (98.5329, 12.6719) (98.3226, 12.4294) knots 0 0 0 0 1 1 1 1
  line L811 (97.4736, 12.1353) -> (96.1879, 12.3855)
  spline S1864 degree 3 poles (93.7488, 20.7255) (93.6711, 20.8324) (93.5771, 20.9264) (93.4702, 21.004) knots 0 0 0 0 1 1 1 1
  spline S1865 degree 3 poles (93.1188, 21.1834) (92.993, 21.2242) (92.8615, 21.2449) (92.7292, 21.2449) knots 0 0 0 0 1 1 1 1
  spline S1866 degree 3 poles (93.4702, 21.004) (93.3632, 21.0819) (93.2447, 21.1424) (93.1188, 21.1834) knots 0 0 0 0 1 1 1 1
  spline S1867 degree 3 poles (93.8175, 15.4437) (94.0285, 15.6864) (94.0939, 16.0233) (93.9891, 16.3273) knots 0 0 0 0 1 1 1 1
  spline S1868 degree 3 poles (91.6807, 15.4008) (91.3655, 15.4626) (91.1071, 15.6877) (91.0027, 15.9914) knots 0 0 0 0 1 1 1 1
  spline S1869 degree 3 poles (70.9848, 20.217) (70.837, 20.2567) (70.6846, 20.2769) (70.5316, 20.277) knots 0 0 0 0 1 1 1 1
  spline S1870 degree 3 poles (68.7818, 18.5267) (68.7819, 18.0626) (68.9663, 17.6176) (69.2945, 17.2895) knots 0 0 0 0 1 1 1 1
  line L812 (91.8677, 17.1836) -> (91.8677, 17.1836)
  line L813 (92.9664, 15.1507) -> (91.6807, 15.4008)
  spline S1871 degree 3 poles (72.2219, 18.9799) (72.1824, 19.1275) (72.1236, 19.2692) (72.0473, 19.4016) knots 0 0 0 0 1 1 1 1
  spline S1872 degree 3 poles (71.4065, 20.0423) (71.2741, 20.1187) (71.1324, 20.1775) (70.9848, 20.217) knots 0 0 0 0 1 1 1 1
  line L814 (32.1334, 28.1096) -> (33.4383, 28.2238)
  spline S1873 degree 3 poles (70.5316, 16.7769) (70.9958, 16.7769) (71.441, 16.9613) (71.7692, 17.2895) knots 0 0 0 0 1 1 1 1
  spline S1874 degree 3 poles (93.8175, 15.4437) (93.6065, 15.2009) (93.2821, 15.0892) (92.9664, 15.1507) knots 0 0 0 0 1 1 1 1
  spline S1875 degree 3 poles (33.4383, 28.2238) (33.7581, 28.2523) (34.0385, 28.449) (34.1741, 28.74) knots 0 0 0 0 1 1 1 1
  spline S1876 degree 3 poles (95.6815, 13.8587) (95.8558, 14.0593) (96.1098, 14.1726) (96.3755, 14.1683) knots 0 0 0 0 1 1 1 1
  spline S1877 degree 3 poles (95.5099, 12.9761) (95.4055, 13.2799) (95.4709, 13.6162) (95.6815, 13.8587) knots 0 0 0 0 1 1 1 1
  line L815 (92.0238, 17.1676) -> (93.31, 16.9175)
  spline S1878 degree 3 poles (31.2394, 29.3865) (31.1034, 29.0951) (31.1332, 28.7534) (31.3175, 28.4899) knots 0 0 0 0 1 1 1 1
  spline S1879 degree 3 poles (72.0473, 19.4016) (71.9708, 19.5341) (71.8774, 19.6561) (71.7692, 19.7643) knots 0 0 0 0 1 1 1 1
  line L816 (33.2817, 30.0169) -> (33.2817, 30.0169)
  line L817 (33.2817, 30.0169) -> (31.9763, 29.9027)
  spline S1880 degree 3 poles (93.9891, 16.3273) (94.0939, 16.0233) (94.0285, 15.6864) (93.8175, 15.4437) knots 0 0 0 0 1 1 1 1
  spline S1881 degree 3 poles (91.0027, 15.9914) (90.8983, 16.2952) (90.9637, 16.6315) (91.1743, 16.8741) knots 0 0 0 0 1 1 1 1
  spline S1882 degree 3 poles (70.5316, 20.277) (70.0676, 20.2769) (69.6226, 20.0925) (69.2945, 19.7643) knots 0 0 0 0 1 1 1 1
  spline S1883 degree 3 poles (69.2945, 19.7643) (68.9662, 19.4361) (68.7818, 18.9909) (68.7818, 18.5267) knots 0 0 0 0 1 1 1 1
  line L818 (70.5316, 20.277) -> (70.5316, 20.277)
  spline S1884 degree 3 poles (26.1545, 30.1461) (26.3388, 29.883) (26.6493, 29.738) (26.9694, 29.7658) knots 0 0 0 0 1 1 1 1
  spline S1885 degree 3 poles (26.0759, 31.0422) (25.9403, 30.7509) (25.9702, 30.4094) (26.1545, 30.1461) knots 0 0 0 0 1 1 1 1
  spline S1886 degree 3 poles (28.2742, 29.88) (28.5941, 29.9085) (28.8745, 30.1052) (29.0101, 30.3962) knots 0 0 0 0 1 1 1 1
  spline S1887 degree 3 poles (29.0101, 30.3962) (29.1459, 30.6874) (29.1162, 31.029) (28.9321, 31.2923) knots 0 0 0 0 1 1 1 1
  spline S1888 degree 3 poles (28.9321, 31.2923) (28.748, 31.5555) (28.4376, 31.7006) (28.1177, 31.6732) knots 0 0 0 0 1 1 1 1
  spline S1889 degree 3 poles (103.5275, 19.1458) (103.6596, 19.1458) (103.7909, 19.125) (103.9166, 19.0843) knots 0 0 0 0 1 1 1 1
  spline S1890 degree 3 poles (17.3684, 49.8953) (17.6047, 49.659) (17.9252, 49.5263) (18.2593, 49.5263) knots 0 0 0 0 1 1 1 1
  spline S1891 degree 3 poles (24.3417, 52.2874) (24.1054, 52.0511) (23.9727, 51.7306) (23.9727, 51.3965) knots 0 0 0 0 1 1 1 1
  spline S1892 degree 3 poles (26.8123, 31.559) (26.4922, 31.5305) (26.2115, 31.3336) (26.0759, 31.0422) knots 0 0 0 0 1 1 1 1
  spline S1893 degree 3 poles (31.9763, 29.9027) (31.6561, 29.8746) (31.3752, 29.6778) (31.2394, 29.3865) knots 0 0 0 0 1 1 1 1
  spline S1894 degree 3 poles (71.7692, 17.2895) (72.0974, 17.6176) (72.2818, 18.0626) (72.2819, 18.5267) knots 0 0 0 0 1 1 1 1
  spline S1895 degree 3 poles (69.2945, 17.2895) (69.6226, 16.9614) (70.0676, 16.777) (70.5316, 16.7769) knots 0 0 0 0 1 1 1 1
  spline S1896 degree 3 poles (31.3175, 28.4899) (31.5019, 28.2264) (31.813, 28.0814) (32.1334, 28.1096) knots 0 0 0 0 1 1 1 1
  spline S1897 degree 3 poles (34.1741, 28.74) (34.3099, 29.0312) (34.2802, 29.3727) (34.0961, 29.6361) knots 0 0 0 0 1 1 1 1
  line L819 (96.3755, 14.1683) -> (96.3755, 14.1683)
  spline S1898 degree 3 poles (34.0961, 29.6361) (33.912, 29.8992) (33.6017, 30.0444) (33.2817, 30.0169) knots 0 0 0 0 1 1 1 1
  line L820 (28.1177, 31.6732) -> (28.1177, 31.6732)
  spline S1899 degree 3 poles (103.9166, 19.0843) (104.0424, 19.0435) (104.161, 18.9831) (104.268, 18.9055) knots 0 0 0 0 1 1 1 1
  spline S1900 degree 3 poles (18.2593, 49.5263) (18.5935, 49.5263) (18.9139, 49.659) (19.1502, 49.8953) knots 0 0 0 0 1 1 1 1
  spline S1901 degree 3 poles (19.5192, 50.7867) (19.5192, 50.9188) (19.4985, 51.0502) (19.4577, 51.1758) knots 0 0 0 0 1 1 1 1
  line L821 (26.9694, 29.7658) -> (28.2742, 29.88)
  line L822 (28.1177, 31.6732) -> (26.8123, 31.559)
  line L823 (19.3513, 51.3841) -> (17.1674, 51.1929)
  spline S1902 degree 3 poles (25.2326, 52.6564) (24.8984, 52.6564) (24.578, 52.5237) (24.3417, 52.2874) knots 0 0 0 0 1 1 1 1
  spline S1903 degree 3 poles (19.4577, 51.1758) (19.4288, 51.2484) (19.3931, 51.3181) (19.3513, 51.3841) knots 0 0 0 0 1 1 1 1
  spline S1904 degree 3 poles (23.9727, 51.3965) (23.9727, 51.0624) (24.1054, 50.7419) (24.3417, 50.5056) knots 0 0 0 0 1 1 1 1
  spline S1905 degree 3 poles (24.3417, 50.5056) (24.578, 50.2693) (24.8984, 50.1366) (25.2326, 50.1366) knots 0 0 0 0 1 1 1 1
  spline S1906 degree 3 poles (25.6217, 50.1981) (25.7475, 50.2389) (25.8661, 50.2993) (25.9731, 50.3769) knots 0 0 0 0 1 1 1 1
  spline S1907 degree 3 poles (19.1502, 49.8953) (19.3866, 50.1317) (19.5194, 50.4524) (19.5192, 50.7867) knots 0 0 0 0 1 1 1 1
  spline S1908 degree 3 poles (25.9731, 50.3769) (26.08, 50.4547) (26.174, 50.5489) (26.2516, 50.656) knots 0 0 0 0 1 1 1 1
  spline S1909 degree 3 poles (72.2819, 18.5267) (72.2818, 18.6797) (72.2616, 18.8321) (72.2219, 18.9799) knots 0 0 0 0 1 1 1 1
  spline S1910 degree 3 poles (25.2326, 50.1366) (25.3647, 50.1366) (25.496, 50.1573) (25.6217, 50.1981) knots 0 0 0 0 1 1 1 1
  spline S1911 degree 3 poles (26.2516, 50.656) (26.3295, 50.763) (26.39, 50.8816) (26.4309, 51.0074) knots 0 0 0 0 1 1 1 1
  spline S1912 degree 3 poles (26.4924, 51.3965) (26.4925, 51.5288) (26.4718, 51.6603) (26.4309, 51.7861) knots 0 0 0 0 1 1 1 1
  spline S1913 degree 3 poles (26.2516, 52.137) (26.174, 52.2441) (26.08, 52.3382) (25.9731, 52.4161) knots 0 0 0 0 1 1 1 1
  spline S1914 degree 3 poles (93.31, 16.9175) (93.6255, 16.8561) (93.8843, 16.6312) (93.9891, 16.3273) knots 0 0 0 0 1 1 1 1
  spline S1915 degree 3 poles (26.4309, 51.0074) (26.4717, 51.1331) (26.4925, 51.2644) (26.4924, 51.3965) knots 0 0 0 0 1 1 1 1
  spline S1916 degree 3 poles (91.1743, 16.8741) (91.3484, 17.0745) (91.6022, 17.1878) (91.8677, 17.1836) knots 0 0 0 0 1 1 1 1
  spline S1917 degree 3 poles (96.1879, 12.3855) (95.8727, 12.4472) (95.6143, 12.6723) (95.5099, 12.9761) knots 0 0 0 0 1 1 1 1
  spline S1918 degree 3 poles (91.8677, 17.1836) (91.9201, 17.1828) (91.9724, 17.1775) (92.0238, 17.1676) knots 0 0 0 0 1 1 1 1
  spline S1919 degree 3 poles (71.7692, 19.7643) (71.661, 19.8725) (71.539, 19.9659) (71.4065, 20.0423) knots 0 0 0 0 1 1 1 1
  spline S1920 degree 3 poles (61.0955, 77.5184) (61.4373, 77.7158) (61.7213, 77.9997) (61.9187, 78.3416) knots 0 0 0 0 1 1 1 1
  spline S1921 degree 3 poles (61.9972, 80.4428) (61.9243, 80.5946) (61.8345, 80.7378) (61.7295, 80.8696) knots 0 0 0 0 1 1 1 1
  spline S1922 degree 3 poles (55.2659, 78.8393) (55.2414, 78.8979) (55.2126, 78.9545) (55.1796, 79.0088) knots 0 0 0 0 1 1 1 1
  spline S1923 degree 3 poles (49.1081, 80.1518) (48.9343, 80.1984) (48.7552, 80.2221) (48.5753, 80.2221) knots 0 0 0 0 1 1 1 1
  spline S1924 degree 3 poles (25.6217, 52.5949) (25.496, 52.6356) (25.3647, 52.6564) (25.2326, 52.6564) knots 0 0 0 0 1 1 1 1
  spline S1925 degree 3 poles (61.373, 43.1257) (61.2414, 43.2308) (61.0983, 43.3207) (60.9466, 43.3939) knots 0 0 0 0 1 1 1 1
  line L824 (59.9705, 43.6166) -> (59.9705, 43.6166)
  spline S1926 degree 3 poles (25.9731, 52.4161) (25.8661, 52.4937) (25.7475, 52.5541) (25.6217, 52.5949) knots 0 0 0 0 1 1 1 1
  spline S1927 degree 3 poles (60.4707, 81.6603) (60.3066, 81.6977) (60.1388, 81.7166) (59.9705, 81.7166) knots 0 0 0 0 1 1 1 1
  spline S1928 degree 3 poles (59.9705, 81.7166) (59.6323, 81.7041) (59.3013, 81.6154) (59.0021, 81.4572) knots 0 0 0 0 1 1 1 1
  spline S1929 degree 3 poles (47.1186, 79.6185) (46.7322, 79.2323) (46.5151, 78.7085) (46.515, 78.1623) knots 0 0 0 0 1 1 1 1
  spline S1930 degree 3 poles (61.0955, 39.4184) (61.4373, 39.6159) (61.7213, 39.8998) (61.9187, 40.2416) knots 0 0 0 0 1 1 1 1
  spline S1931 degree 3 poles (58.8455, 39.4184) (59.1875, 39.2208) (59.5755, 39.1167) (59.9705, 39.1166) knots 0 0 0 0 1 1 1 1
  spline S1932 degree 3 poles (62.2205, 41.3666) (62.2203, 41.5351) (62.2013, 41.7031) (62.1636, 41.8674) knots 0 0 0 0 1 1 1 1
  spline S1933 degree 3 poles (57.7205, 41.3666) (57.7204, 40.9717) (57.8243, 40.5837) (58.0218, 40.2416) knots 0 0 0 0 1 1 1 1
  spline S1934 degree 3 poles (60.9466, 43.3939) (60.7947, 43.467) (60.6351, 43.5228) (60.4707, 43.5603) knots 0 0 0 0 1 1 1 1
  spline S1935 degree 3 poles (62.1636, 79.9674) (62.1261, 80.1316) (62.0703, 80.291) (61.9972, 80.4428) knots 0 0 0 0 1 1 1 1
  spline S1936 degree 3 poles (60.4707, 43.5603) (60.3066, 43.5977) (60.1388, 43.6166) (59.9705, 43.6166) knots 0 0 0 0 1 1 1 1
  spline S1937 degree 3 poles (26.4309, 51.7861) (26.3899, 51.9118) (26.3294, 52.0302) (26.2516, 52.137) knots 0 0 0 0 1 1 1 1
  spline S1938 degree 3 poles (62.2205, 79.4666) (62.2203, 79.6351) (62.2013, 79.8031) (62.1636, 79.9674) knots 0 0 0 0 1 1 1 1
  spline S1939 degree 3 poles (52.8076, 78.4501) (52.8076, 78.116) (52.9403, 77.7955) (53.1766, 77.5592) knots 0 0 0 0 1 1 1 1
  spline S1940 degree 3 poles (55.3274, 78.4501) (55.3274, 78.5823) (55.3066, 78.7136) (55.2659, 78.8393) knots 0 0 0 0 1 1 1 1
  spline S1941 degree 3 poles (50.0099, 79.6351) (49.8884, 79.7551) (49.7525, 79.8596) (49.6052, 79.9462) knots 0 0 0 0 1 1 1 1
  spline S1942 degree 3 poles (47.1186, 76.7055) (47.5049, 76.3191) (48.0289, 76.102) (48.5753, 76.102) knots 0 0 0 0 1 1 1 1
  spline S1943 degree 3 poles (49.1081, 76.1722) (49.2821, 76.2188) (49.4492, 76.2879) (49.6052, 76.3779) knots 0 0 0 0 1 1 1 1
  spline S1944 degree 3 poles (49.6052, 79.9462) (49.4492, 80.0362) (49.2821, 80.1053) (49.1081, 80.1518) knots 0 0 0 0 1 1 1 1
  spline S1945 degree 3 poles (48.5753, 76.102) (48.7552, 76.102) (48.9343, 76.1256) (49.1081, 76.1722) knots 0 0 0 0 1 1 1 1
  spline S1946 degree 3 poles (52.9916, 78.894) (52.9023, 78.7592) (52.8399, 78.6085) (52.8076, 78.4501) knots 0 0 0 0 1 1 1 1
  spline S1947 degree 3 poles (50.0316, 76.7055) (50.1589, 76.8327) (50.2691, 76.9761) (50.3592, 77.1319) knots 0 0 0 0 1 1 1 1
  spline S1948 degree 3 poles (59.9705, 39.1166) (60.3655, 39.1167) (60.7535, 39.2208) (61.0955, 39.4184) knots 0 0 0 0 1 1 1 1
  spline S1949 degree 3 poles (54.0675, 77.1897) (54.4017, 77.1899) (54.7222, 77.3228) (54.9584, 77.5592) knots 0 0 0 0 1 1 1 1
  spline S1950 degree 3 poles (57.7205, 79.4666) (57.7204, 79.0717) (57.8243, 78.6837) (58.0218, 78.3416) knots 0 0 0 0 1 1 1 1
  spline S1951 degree 3 poles (58.8455, 77.5184) (59.1875, 77.3208) (59.5755, 77.2167) (59.9705, 77.2166) knots 0 0 0 0 1 1 1 1
  spline S1952 degree 3 poles (58.8455, 43.3153) (58.5034, 43.1178) (58.2193, 42.8337) (58.0218, 42.4916) knots 0 0 0 0 1 1 1 1
  spline S1953 degree 3 poles (53.1766, 77.5592) (53.4128, 77.3228) (53.7333, 77.1899) (54.0675, 77.1897) knots 0 0 0 0 1 1 1 1
  spline S1954 degree 3 poles (46.515, 78.1623) (46.515, 77.6159) (46.7321, 77.0919) (47.1186, 76.7055) knots 0 0 0 0 1 1 1 1
  spline S1955 degree 3 poles (60.9466, 81.4939) (60.7947, 81.567) (60.6351, 81.6228) (60.4707, 81.6603) knots 0 0 0 0 1 1 1 1
  spline S1956 degree 3 poles (62.1636, 41.8674) (62.1262, 42.0317) (62.0704, 42.1914) (61.9972, 42.3433) knots 0 0 0 0 1 1 1 1
  spline S1957 degree 3 poles (61.9972, 42.3433) (61.9242, 42.495) (61.8344, 42.638) (61.7295, 42.7696) knots 0 0 0 0 1 1 1 1
  spline S1958 degree 3 poles (58.0218, 78.3416) (58.2193, 77.9997) (58.5034, 77.7158) (58.8455, 77.5184) knots 0 0 0 0 1 1 1 1
  spline S1959 degree 3 poles (48.5753, 80.2221) (48.0289, 80.2221) (47.5049, 80.005) (47.1186, 79.6185) knots 0 0 0 0 1 1 1 1
  spline S1960 degree 3 poles (49.6052, 76.3779) (49.761, 76.468) (49.9044, 76.5782) (50.0316, 76.7055) knots 0 0 0 0 1 1 1 1
  spline S1961 degree 3 poles (61.9187, 78.3416) (62.1163, 78.6836) (62.2204, 79.0716) (62.2205, 79.4666) knots 0 0 0 0 1 1 1 1
  spline S1962 degree 3 poles (61.7295, 80.8696) (61.6244, 81.0013) (61.5048, 81.1207) (61.373, 81.2257) knots 0 0 0 0 1 1 1 1
  spline S1963 degree 3 poles (58.0218, 42.4916) (57.8243, 42.1496) (57.7204, 41.7616) (57.7205, 41.3666) knots 0 0 0 0 1 1 1 1
  line L825 (25.2326, 52.6564) -> (25.2326, 52.6564)
  line L826 (59.0021, 81.4572) -> (59.0698, 80.1642)
  spline S1964 degree 3 poles (54.9584, 77.5592) (55.1946, 77.7955) (55.3274, 78.116) (55.3274, 78.4501) knots 0 0 0 0 1 1 1 1
  spline S1965 degree 3 poles (50.3592, 77.1319) (50.4492, 77.2879) (50.5183, 77.455) (50.5649, 77.629) knots 0 0 0 0 1 1 1 1
  spline S1966 degree 3 poles (50.5649, 77.629) (50.6115, 77.8029) (50.6351, 77.9822) (50.6351, 78.1623) knots 0 0 0 0 1 1 1 1
  spline S1967 degree 3 poles (43.0826, 79.1343) (42.7485, 79.1343) (42.428, 79.0016) (42.1917, 78.7654) knots 0 0 0 0 1 1 1 1
  line L827 (50.5359, 78.7654) -> (50.0569, 78.7406)
  line L828 (50.0569, 78.7406) -> (50.0099, 79.6351)
  line L829 (59.0698, 80.1642) -> (57.8905, 80.1022)
  spline S1968 degree 3 poles (59.9705, 43.6166) (59.5755, 43.6167) (59.1875, 43.5128) (58.8455, 43.3153) knots 0 0 0 0 1 1 1 1
  spline S1969 degree 3 poles (58.0218, 40.2416) (58.2193, 39.8997) (58.5034, 39.6158) (58.8455, 39.4184) knots 0 0 0 0 1 1 1 1
  line L830 (55.1796, 79.0088) -> (52.9916, 78.894)
  spline S1970 degree 3 poles (59.9705, 77.2166) (60.3655, 77.2167) (60.7535, 77.3208) (61.0955, 77.5184) knots 0 0 0 0 1 1 1 1
  spline S1971 degree 3 poles (50.6351, 78.1623) (50.6351, 78.3422) (50.6114, 78.5213) (50.5649, 78.6951) knots 0 0 0 0 1 1 1 1
  spline S1972 degree 3 poles (50.5649, 78.6951) (50.5556, 78.7187) (50.546, 78.7421) (50.5359, 78.7654) knots 0 0 0 0 1 1 1 1
  spline S1973 degree 3 poles (61.7295, 42.7696) (61.6244, 42.9013) (61.5048, 43.0207) (61.373, 43.1257) knots 0 0 0 0 1 1 1 1
  spline S1974 degree 3 poles (61.9187, 40.2416) (62.1163, 40.5836) (62.2204, 40.9716) (62.2205, 41.3666) knots 0 0 0 0 1 1 1 1
  spline S1975 degree 3 poles (61.373, 81.2257) (61.2414, 81.3307) (61.0983, 81.4207) (60.9466, 81.4939) knots 0 0 0 0 1 1 1 1
  spline S1976 degree 3 poles (57.8905, 80.1022) (57.803, 79.8998) (57.7457, 79.6857) (57.7205, 79.4666) knots 0 0 0 0 1 1 1 1
  spline S1977 degree 3 poles (82.7758, 44.5995) (82.9081, 44.5996) (83.0396, 44.5788) (83.1654, 44.538) knots 0 0 0 0 1 1 1 1
  spline S1978 degree 3 poles (83.7954, 44.0802) (83.873, 43.9731) (83.9334, 43.8545) (83.9742, 43.7287) knots 0 0 0 0 1 1 1 1
  spline S1979 degree 3 poles (48.2947, 44.2088) (48.2946, 43.6625) (48.5115, 43.1385) (48.8978, 42.7521) knots 0 0 0 0 1 1 1 1
  spline S1980 degree 3 poles (62.1636, 41.8674) (62.2013, 41.7031) (62.2203, 41.5351) (62.2205, 41.3666) knots 0 0 0 0 1 1 1 1
  spline S1981 degree 3 poles (41.8228, 77.8745) (41.8227, 77.5403) (41.9555, 77.2199) (42.1917, 76.9836) knots 0 0 0 0 1 1 1 1
  line L831 (14.241, 50.9366) -> (14.1635, 51.8202)
  spline S1982 degree 3 poles (56.2363, 45.695) (56.1107, 45.7358) (55.9793, 45.7566) (55.8472, 45.7565) knots 0 0 0 0 1 1 1 1
  spline S1983 degree 3 poles (50.3545, 42.1485) (50.5346, 42.1485) (50.7139, 42.1721) (50.8878, 42.2188) knots 0 0 0 0 1 1 1 1
  spline S1984 degree 3 poles (55.8472, 45.7565) (55.9793, 45.7566) (56.1107, 45.7358) (56.2363, 45.695) knots 0 0 0 0 1 1 1 1
  spline S1985 degree 3 poles (57.0456, 44.8858) (57.0864, 44.7601) (57.1071, 44.6288) (57.1071, 44.4967) knots 0 0 0 0 1 1 1 1
  spline S1986 degree 3 poles (56.2363, 45.695) (56.3622, 45.6541) (56.4808, 45.5936) (56.5877, 45.5157) knots 0 0 0 0 1 1 1 1
  spline S1987 degree 3 poles (54.9563, 43.6058) (54.7199, 43.842) (54.587, 44.1624) (54.5868, 44.4967) knots 0 0 0 0 1 1 1 1
  spline S1988 degree 3 poles (48.8978, 42.7521) (49.2841, 42.3656) (49.8081, 42.1485) (50.3545, 42.1485) knots 0 0 0 0 1 1 1 1
  spline S1989 degree 3 poles (48.8978, 45.6656) (48.5115, 45.2792) (48.2946, 44.7552) (48.2947, 44.2088) knots 0 0 0 0 1 1 1 1
  spline S1990 degree 3 poles (50.8878, 42.2188) (51.0617, 42.2655) (51.2286, 42.3348) (51.3844, 42.425) knots 0 0 0 0 1 1 1 1
  spline S1991 degree 3 poles (56.5877, 45.5157) (56.6946, 45.4381) (56.7886, 45.3441) (56.8663, 45.2372) knots 0 0 0 0 1 1 1 1
  spline S1992 degree 3 poles (56.8663, 45.2372) (56.9441, 45.1302) (57.0046, 45.0116) (57.0456, 44.8858) knots 0 0 0 0 1 1 1 1
  spline S1993 degree 3 poles (17.1674, 51.1929) (17.0879, 51.0684) (17.0309, 50.9309) (16.999, 50.7867) knots 0 0 0 0 1 1 1 1
  spline S1994 degree 3 poles (54.5868, 44.4967) (54.587, 44.8309) (54.7199, 45.1514) (54.9563, 45.3876) knots 0 0 0 0 1 1 1 1
  spline S1995 degree 3 poles (63.6405, 41.9935) (63.4797, 42.272) (63.4797, 42.6151) (63.6405, 42.8937) knots 0 0 0 0 1 1 1 1
  spline S1996 degree 3 poles (16.999, 50.7867) (16.999, 50.4523) (17.1319, 50.1316) (17.3684, 49.8953) knots 0 0 0 0 1 1 1 1
  line L832 (14.7128, 50.9779) -> (14.241, 50.9366)
  spline S1997 degree 3 poles (62.2205, 41.3666) (62.2204, 40.9716) (62.1163, 40.5836) (61.9187, 40.2416) knots 0 0 0 0 1 1 1 1
  spline S1998 degree 3 poles (43.0826, 76.6141) (43.4168, 76.6142) (43.7373, 76.7471) (43.9735, 76.9836) knots 0 0 0 0 1 1 1 1